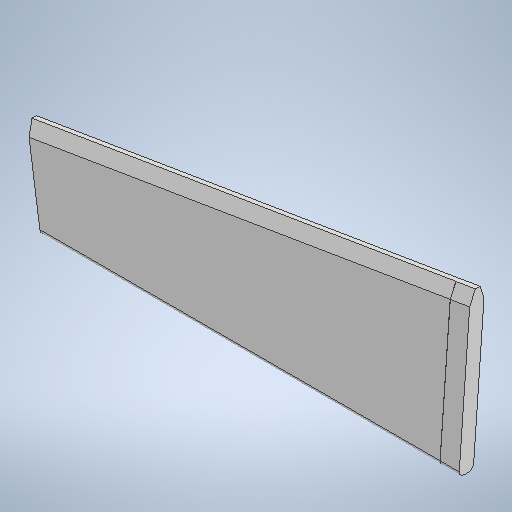
# Autodesk Inventor part: vertical_stabilizer_01
Saved by Autodesk Inventor 2025.3 (Build 293356000, 356)
## iProperties
Created: 2025-07-09
Part Number: vertical_stabilizer_01
Material: Generic
Document SubType Name: Modeling
Designer: steve
Density: 1 g/cm^3
Appearance: Default
Author: steve
Autodesk Inventor part; units mm, degrees
ref_plane "YZ Plane" through (0, 0, 0) normal (1, 0, 0) x (0, 1, 0)
ref_plane "XZ Plane" through (0, 0, 0) normal (0, 1, 0) x (-1, 0, 0)
ref_plane "XY Plane" through (0, 0, 0) normal (0, 0, 1) x (1, 0, 0)
sketch "Sketch1" plane through (0, 0, 0) normal (0, 0, 1) x (1, 0, 0)
  line L0 (-47.7435, -77.7913) -> (102.2565, -77.7913)
  line L1 (102.2565, -77.7913) -> (109.4965, -77.7913)
  line L2 (-47.7435, -77.7913) -> (-47.7435, -13.2313) construction
  line L3 (-47.7435, -13.2313) -> (-47.7435, 15.6487) construction
  line L4 (-47.7435, -77.7913) -> (-47.7435, -72.7913)
  line L5 (-47.7435, -72.7913) -> (-61.2235, -72.7913) construction
  line L6 (-47.7435, -72.7913) -> (-47.7435, -57.7913) construction
  line L7 (-47.7435, -57.7913) -> (-65.2735, -57.7913) construction
  line L8 (-47.7435, -57.7913) -> (-47.7435, -42.7913) construction
  line L9 (-47.7435, -42.7913) -> (-67.4235, -42.7913) construction
  line L10 (-47.7435, -42.7913) -> (-47.7435, -27.7913) construction
  line L11 (-47.7435, -27.7913) -> (-69.5835, -27.7913) construction
  line L12 (-47.7435, -27.7913) -> (-47.7435, -12.7913) construction
  line L13 (-47.7435, -12.7913) -> (-72.3735, -12.7913) construction
  line L14 (-47.7435, -77.7913) -> (42.2565, -77.7913)
  line L15 (42.2565, -77.7913) -> (42.2565, 92.2087) construction
  line L16 (42.2565, 92.2087) -> (-47.7435, 15.6487)
  line L17 (42.2565, 92.2087) -> (47.8065, 92.2087)
  line L18 (42.2565, -77.7913) -> (67.2565, -77.7913)
  line L19 (67.2565, -77.7913) -> (67.2565, -22.7913) construction
  line L20 (67.2565, -22.7913) -> (63.6956, -23.3847)
  line L21 (102.2565, -77.7913) -> (97.2565, -77.7913)
  line L22 (97.2565, -77.7913) -> (97.2565, -17.7913) construction
  line L23 (97.2565, -17.7913) -> (113.897, -15.0179)
  line L24 (109.4965, -77.7913) -> (113.897, -15.0179)
  line L25 (97.2565, -17.7913) -> (67.2565, -22.7913)
  line L26 (63.6956, -23.3847) -> (47.8065, 92.2087)
  spline S0 degree 2 poles (42.2565, 92.2087) (45.0586, 96.9623) (47.8065, 92.2087) knots 0 0 0 1 1 1
  line L27 (-59.7435, -93.9838) -> (-59.7435, 5.4407) construction
  line L28 (-47.7435, 15.6487) -> (-59.7435, 5.4407)
  line L29 (-59.7435, 5.4407) -> (-47.7435, -77.7913)
  line L30 (-69.5835, -27.7913) -> (-65.2735, -57.7913)
  line L31 (-47.7435, -77.7913) -> (-61.2235, -72.7913) construction
  line L32 (-61.2235, -72.7913) -> (-65.2735, -57.7913) construction
  spline S1 degree 2 poles (-47.7435, -77.7913) (-61.2235, -72.7913) (-65.2735, -57.7913) knots 1 1 1 2 2 2
  line L33 (-69.5835, -27.7913) -> (-72.3735, -12.7913) construction
  line L34 (-72.3735, -12.7913) -> (-59.7435, 5.4407) construction
  spline S2 degree 2 poles (-69.5835, -27.7913) (-72.3735, -12.7913) (-59.7435, 5.4407) knots 1 1 1 2 2 2
  line L35 (102.2565, -77.7913) -> (106.5714, -16.2388)
  line L36 (63.6956, -23.3847) -> (-52.7885, -42.7988)
  line L37 (-131.9637, -55.9946) -> (-133.7071, -56.2852)
  point P0 (0, 0)
  point P1 (45.0505, 94.5855)
  point P2 (-53.7435, 10.5447)
  dimension "d0" = 150
  dimension "d1" = 7.24
  dimension "d2" = 64.56
  dimension "d3" = 28.88
  dimension "d4" = 13.48
  dimension "d5" = 15
  dimension "d6" = 17.53
  dimension "d7" = 15
  dimension "d8" = 19.68
  dimension "d9" = 15
  dimension "d10" = 21.84
  dimension "d11" = 15
  dimension "d12" = 24.63
  dimension "d13" = 90
  dimension "d14" = 170
  dimension "d15" = 5.55
  dimension "d16" = 25
  dimension "d17" = 55
  dimension "d18" = 3.61
  dimension "d19" = 5
  dimension "d20" = 60
  dimension "d21" = 16.87
  dimension "d22" = 12
  dimension "d23" = 5
  constraints: 68 end point, 16 point on line, 9 perpendicular, 5 collinear, 2 coincident, 2 vertical, 1 horizontal, 1 midpoint, 1 parallel, 9 other
  measures "d0" distance of L0.start L0.end
  measures "d1" distance of L0.end L24.start
  measures "d2" distance of L0.start L3.start
  measures "d3" distance of L3.start L16.end
  measures "d4" distance of L6.start L5.end
  measures "d5" distance of L6.start L7.start
  measures "d6" distance of L7.start L30.end
  measures "d7" distance of L7.start L9.start
  measures "d8" distance of L9.start L9.end
  measures "d9" distance of L9.start L11.start
  measures "d10" distance of L11.start L11.end
  measures "d11" distance of L11.start L12.end
  measures "d12" distance of L12.end L13.end
  measures "d13" distance of L0.start L14.end
  measures "d14" distance of L14.end L15.end
  measures "d15" distance of L15.end L26.end
  measures "d16" distance of L14.end L18.end
  measures "d17" distance of L18.end L20.start
  measures "d18" distance of L20.start L36.start
  measures "d19" distance of L0.end L22.start
  measures "d20" distance of L22.start L25.start
  measures "d21" distance of L23.end L25.start
  measures "d22" distance between parallel lines of L27 L3
  measures "d23" distance of L0.start L6.start
extrude "Extrusion1" add sketch "Sketch1" along normal mid plane 5.3 contours L29 L36 L20 L25 L23 L35 L0
extrude "Extrusion2" add sketch "Sketch1" along normal mid plane 5.4 contours L35 L23 L24 L1
chamfer "Chamfer1" distance 5 angle 20 1 edges at (26.8914, -29.5188, 2.65) measured on face at (52.0131, -45.6096, 2.65)
chamfer "Chamfer2" distance 5 angle 20 1 edges at (110.2342, -15.6283, 2.7) measured on face at (109.9883, -36.3493, 2.7)
chamfer "Chamfer3" distance 5 angle 20 1 edges at (26.8914, -29.5188, -2.65) measured on face at (52.0131, -45.6096, -2.65)
chamfer "Chamfer4" distance 5 angle 20 1 edges at (110.2342, -15.6283, -2.7) measured on face at (109.9883, -36.3493, -2.7)
fillet "Fillet1" radius 2 4 edges at (27.2565, -77.7913, -2.65) (105.8765, -77.7913, -2.7) (27.2565, -77.7913, 2.65) (105.8765, -77.7913, 2.7)
body "Solid1"
